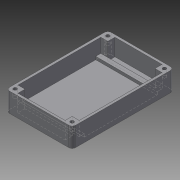
# Autodesk Inventor part: base v2
Saved by Autodesk Inventor 2015 (Build 190159000, 159)
## iProperties
Created: 2020-03-18
Part Number: base v2
Material: Generic
Document SubType Name: Modeling
Designer: Toby
Density: 1 g/cm^3
Appearance: Default
Author: Toby
Autodesk Inventor part; units mm, degrees
ref_plane "YZ Plane" through (0, 0, 0) normal (1, 0, 0) x (0, 1, 0)
ref_plane "XZ Plane" through (0, 0, 0) normal (0, 1, 0) x (-1, 0, 0)
ref_plane "XY Plane" through (0, 0, 0) normal (0, 0, 1) x (1, 0, 0)
sketch "Sketch1" plane through (0, 0, 0) normal (0, 0, 1) x (1, 0, 0)
  line L0 (-34.1779, 55.6594) -> (21.8221, 55.6594)
  line L1 (21.8221, 55.6594) -> (21.8221, -30.6406)
  line L2 (21.8221, -30.6406) -> (-34.1779, -30.6406)
  line L3 (-34.1779, -30.6406) -> (-34.1779, 55.6594)
  point P0 (0, 0)
  dimension "d0" = 56
  dimension "d1" = 86.3
  constraints: 8 end point, 2 parallel, 1 horizontal, 1 perpendicular
  measures "d0" distance between parallel lines of L1 L3
  measures "d1" distance between parallel lines of L2 L0
extrude "Extrusion1" add sketch "Sketch1" along normal blind 2
sketch "Sketch2" plane through (0, 0, 2) normal (0, 0, 1) x (1, 0, 0)
  line L0 (-34.1779, 55.6594) -> (21.8221, 55.6594)
  line L1 (21.8221, 55.6594) -> (21.8221, -30.6406)
  line L2 (21.8221, -30.6406) -> (-34.1779, -30.6406)
  line L3 (-34.1779, -30.6406) -> (-34.1779, 55.6594)
  line L4 (-32.1779, 53.6594) -> (19.8221, 53.6594)
  line L5 (19.8221, 53.6594) -> (19.8221, -28.6406)
  line L6 (19.8221, -28.6406) -> (-32.1779, -28.6406)
  line L7 (-32.1779, -28.6406) -> (-32.1779, 53.6594)
  point P0 (0, 0)
  dimension "d4" = 2
  dimension "d5" = 2
  dimension "d6" = 2
  dimension "d7" = 2
  constraints: 16 end point, 4 parallel, 2 horizontal, 2 perpendicular
  measures "d4" distance between parallel lines of L4 L0
  measures "d5" distance between parallel lines of L2 L6
  measures "d6" distance between parallel lines of L3 L7
  measures "d7" distance between parallel lines of L1 L5
extrude "Extrusion2" add sketch "Sketch2" along normal blind 14.4
sketch "Sketch3" plane through (0, 0, 2) normal (0, 0, 1) x (1, 0, 0)
  line L0 (-34.1779, 55.6594) -> (-26.1779, 55.6594)
  line L1 (-26.1779, 55.6594) -> (-26.1779, 47.6594)
  line L2 (-26.1779, 47.6594) -> (-34.1779, 47.6594)
  line L3 (-34.1779, 47.6594) -> (-34.1779, 55.6594)
  line L4 (21.8221, 55.6594) -> (13.8221, 55.6594)
  line L5 (13.8221, 55.6594) -> (13.8221, 47.6594)
  line L6 (13.8221, 47.6594) -> (21.8221, 47.6594)
  line L7 (21.8221, 47.6594) -> (21.8221, 55.6594)
  line L8 (-34.1779, -30.6406) -> (-26.1779, -30.6406)
  line L9 (-26.1779, -30.6406) -> (-26.1779, -22.6406)
  line L10 (-26.1779, -22.6406) -> (-34.1779, -22.6406)
  line L11 (-34.1779, -22.6406) -> (-34.1779, -30.6406)
  line L12 (21.8221, -30.6406) -> (13.8221, -30.6406)
  line L13 (13.8221, -30.6406) -> (13.8221, -22.6406)
  line L14 (13.8221, -22.6406) -> (21.8221, -22.6406)
  line L15 (21.8221, -22.6406) -> (21.8221, -30.6406)
  line L16 (-34.1779, -30.6406) -> (21.8221, -30.6406) projected
  point P0 (0, 0)
  dimension "d10" = 8
  dimension "d11" = 8
  dimension "d12" = 8
  dimension "d13" = 8
  dimension "d14" = 8
  dimension "d15" = 8
  dimension "d16" = 8
  dimension "d17" = 8
  constraints: 32 end point, 8 parallel, 4 horizontal, 4 perpendicular, 1 collinear, 1 point on line
  measures "d10" distance of L1.end L2.end
  measures "d11" distance of L0.end L1.end
  measures "d12" distance of L6.end L5.end
  measures "d13" distance of L5.end L4.end
  measures "d14" distance of L10.end L9.end
  measures "d15" distance of L9.end L8.end
  measures "d16" distance of L13.end L14.end
  measures "d17" distance of L12.end L13.end
extrude "Extrusion3" add sketch "Sketch3" along normal blind 14.4
sketch "Sketch4" plane through (0, 0, 16.4) normal (0, 0, 1) x (1, 0, 0)
  line L0 (-26.1779, -22.6406) -> (-32.1779, -22.6406) projected
  line L1 (19.8221, -22.6406) -> (13.8221, -22.6406) projected
  line L2 (21.8221, 55.6594) -> (21.8221, -30.6406) projected
  line L3 (21.8221, 55.6594) -> (-34.1779, 55.6594) projected
  line L4 (-34.1779, -30.6406) -> (-34.1779, 55.6594) projected
  point P0 (0, 0)
  point P1 (-30.1779, 51.6594)
  point P2 (17.8221, 51.6594)
  point P3 (-30.5754, -26.6406)
  point P4 (17.8221, -26.6406)
  dimension "d20" = 4
  dimension "d21" = 4
  dimension "d22" = 4
  dimension "d23" = 4
  dimension "d24" = 4
  dimension "d25" = 4
  dimension "d26" = 4
  measures "d20" distance from line of L0 point (-30.575, -26.641)
  measures "d21" distance from line of L1 point (17.822, -26.641)
  measures "d22" distance from line of L2 point (17.822, -26.641)
  measures "d23" distance from line of L3 point (-30.178, 51.659)
  measures "d24" distance from line of L4 point (-30.178, 51.659)
  measures "d25" distance from line of L3 point (17.822, 51.659)
  measures "d26" distance from line of L2 point (17.822, 51.659)
hole "Hole1" at (-30.1779, 51.6594, 16.4) at (17.8221, 51.6594, 16.4) at (-30.5754, -26.6406, 16.4) at (17.8221, -26.6406, 16.4) direction (0, 0, -1) diameter 3 depth 6 tip angle 118
fillet "Fillet1" radius 3 4 edges at (-34.1779, 55.6594, 8.2) (21.8221, 55.6594, 8.2) (-34.1779, -30.6406, 8.2) (21.8221, -30.6406, 8.2)
sketch "Sketch5" plane through (0, 0, 2) normal (0, 0, 1) x (1, 0, 0)
  line L0 (-32.1779, 47.6594) -> (19.8221, 47.6594)
  line L1 (19.8221, 47.6594) -> (19.8221, 43.3594)
  line L2 (19.8221, 43.3594) -> (-32.1779, 43.3594)
  line L3 (-32.1779, 43.3594) -> (-32.1779, 47.6594)
  line L4 (19.8221, 47.6594) -> (19.8221, -22.6406) projected
  line L5 (-32.1779, -22.6406) -> (19.8221, -22.6406)
  line L6 (19.8221, -22.6406) -> (19.8221, -18.3406)
  line L7 (19.8221, -18.3406) -> (-32.1779, -18.3406)
  line L8 (-32.1779, -18.3406) -> (-32.1779, -22.6406)
  point P0 (0, 0)
  dimension "d35" = 4.3
  dimension "d36" = 4.3
  constraints: 16 end point, 4 parallel, 2 horizontal, 2 perpendicular, 1 collinear, 1 point on line
  measures "d35" distance between parallel lines of L0 L2
  measures "d36" distance between parallel lines of L5 L7
extrude "Extrusion4" add sketch "Sketch5" along normal blind 2.5
body "Solid1"
